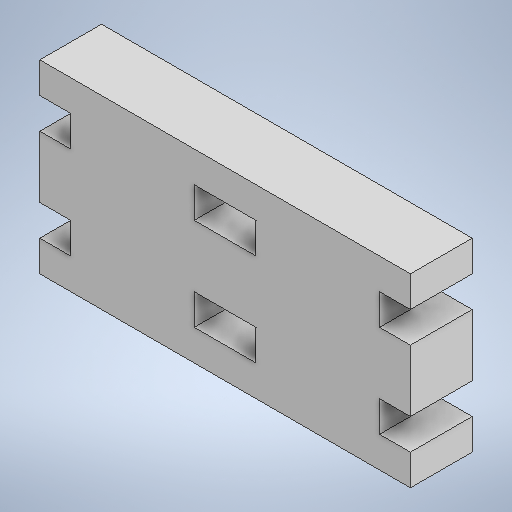
# Autodesk Inventor part: Base
Saved by Autodesk Inventor 2025.1 (Build 291241020, 241B)
## iProperties
Created: 2024-10-29
Part Number: Base
Material: Generic
Document SubType Name: Modeling
Designer: jjk
Density: 1 g/cm^3
Appearance: Default
Author: jjk
Autodesk Inventor part; units mm, degrees
ref_plane "YZ Plane" through (0, 0, 0) normal (1, 0, 0) x (0, 1, 0)
ref_plane "XZ Plane" through (0, 0, 0) normal (0, 1, 0) x (-1, 0, 0)
ref_plane "XY Plane" through (0, 0, 0) normal (0, 0, 1) x (1, 0, 0)
sketch "Sketch1" plane through (0, 0, 0) normal (0, 0, 1) x (1, 0, 0)
  line L0 (152.4, 12.7) -> (152.4, 76.2)
  line L1 (0, 76.2) -> (0, 0)
  line L2 (0, 76.2) -> (12.7, 76.2)
  line L3 (12.7, 76.2) -> (12.7, 63.5)
  line L4 (12.7, 63.5) -> (0, 63.5)
  line L5 (0, 63.5) -> (0, 76.2)
  line L6 (152.4, 76.2) -> (139.7, 76.2)
  line L7 (139.7, 76.2) -> (139.7, 63.5)
  line L8 (139.7, 63.5) -> (152.4, 63.5)
  line L9 (152.4, 63.5) -> (152.4, 76.2)
  line L10 (63.5, 76.2) -> (88.9, 76.2)
  line L11 (88.9, 76.2) -> (88.9, 63.5)
  line L12 (88.9, 63.5) -> (63.5, 63.5)
  line L13 (63.5, 63.5) -> (63.5, 76.2)
  line L14 (152.4, 76.2) -> (152.4, 88.9)
  line L15 (152.4, 88.9) -> (0, 88.9)
  line L16 (0, 88.9) -> (0, 76.2)
  line L17 (12.7, 38.1) -> (12.7, 25.4)
  line L18 (12.7, 25.4) -> (0, 25.4)
  line L19 (0, 25.4) -> (0, 38.1)
  line L20 (0, 38.1) -> (12.7, 38.1)
  line L21 (88.9, 25.4) -> (63.5, 25.4)
  line L22 (63.5, 25.4) -> (63.5, 38.1)
  line L23 (88.9, 38.1) -> (88.9, 25.4)
  line L24 (63.5, 38.1) -> (88.9, 38.1)
  line L25 (139.7, 38.1) -> (139.7, 25.4)
  line L26 (139.7, 25.4) -> (152.4, 25.4)
  line L27 (152.4, 25.4) -> (152.4, 38.1)
  line L28 (152.4, 38.1) -> (139.7, 38.1)
  line L29 (0, 76.2) -> (12.7, 76.2)
  line L30 (12.7, 76.2) -> (0, 76.2)
  line L31 (152.4, 76.2) -> (139.7, 76.2)
  line L32 (88.9, 76.2) -> (63.5, 76.2)
  line L33 (63.5, 76.2) -> (88.9, 76.2)
  line L34 (139.7, 76.2) -> (152.4, 76.2)
  line L35 (0, 12.7) -> (152.4, 12.7)
  point P0 (146.05, 76.2)
  point P1 (76.2, 76.2)
  point P2 (76.2, 38.1)
  point P3 (146.05, 38.1)
  point P4 (6.35, 25.4)
  point P5 (0, 63.5)
  point P6 (0, 25.4)
  dimension "d0" = 152.4
  dimension "d2" = 12.7
  dimension "d4" = 12.7
  dimension "d5" = 12.7
  dimension "d6" = 63.5
  dimension "d7" = 25.4
  dimension "d8" = 12.7
  dimension "d12" = 38.1
  dimension "d18" = 12.7
  dimension "d19" = 12.7
  dimension "d20" = 12.7
  constraints: 72 end point, 11 parallel, 7 perpendicular, 6 horizontal, 3 midpoint, 1 point on line, 1 vertical, 26 other
  measures "d0" distance between parallel lines of L1 L0
  measures "d2" distance between parallel lines of L1 L3
  measures "d4" distance between parallel lines of L0 L7
  measures "d5" distance from line of point (146.05, 76.2) L8
  measures "d6" distance between parallel lines of L1 L13
  measures "d7" distance between parallel lines of L11 L13
  measures "d8" distance from line of point (76.2, 76.2) L12
  measures "d12" distance of L2.end L17.start
  measures "d18" distance between parallel lines of L15 L10
  measures "d19" distance from line of L35 point (6.35, 25.4)
  measures "d20" distance between parallel lines of L35 L21
extrude "Extrusion1" add sketch "Sketch1" along normal blind 25.4 contours L35 L1 L18 L17 L20 L4 L3 L2 L16 L15 L14 L6 L7 L8 L0 L28 L25 L26
body "Solid1"
